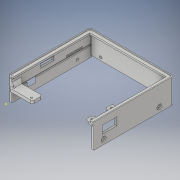
# Autodesk Inventor part: Screen_Top_Open_Back
Saved by Autodesk Inventor 2019 (Build 230136000, 136)
## iProperties
Created: 2020-02-14
Part Number: Screen_Top_Open_Back
Material: Generic
Document SubType Name: Modeling
Designer: zhang
Density: 1 g/cm^3
Appearance: Default
Author: zhang
Autodesk Inventor part; units mm, degrees
note: some values were not read from the file. Chosen so that the rebuilt part matches the saved one: edges of "Chamfer4".
ref_plane "YZ Plane" through (0, 0, 0) normal (1, 0, 0) x (0, 1, 0)
ref_plane "XZ Plane" through (0, 0, 0) normal (0, 1, 0) x (-1, 0, 0)
ref_plane "XY Plane" through (0, 0, 0) normal (0, 0, 1) x (1, 0, 0)
sketch "Sketch1" plane through (0, 0, 0) normal (0, 1, 0) x (-1, 0, 0)
  line L0 (-3, 0) -> (-83, 0)
  line L1 (-86, -3) -> (-86, -83)
  line L2 (-83, -86) -> (-3, -86)
  line L3 (0, -83) -> (0, -3)
  arc A0 (-3, -86) -> (0, -83) centre (-3, -83) ccw
  arc A1 (-86, -83) -> (-83, -86) centre (-83, -83) ccw
  arc A2 (0, -3) -> (-3, 0) centre (-3, -3) ccw
  arc A3 (-83, 0) -> (-86, -3) centre (-83, -3) ccw
  point P0 (0, 0)
  point P1 (-86, -86)
  point P2 (-86, 0)
  point P3 (0, -86)
  dimension "d0" = 86
  dimension "d1" = 86
  dimension "d4" = 3
  constraints: 8 end point, 8 point on circle, 8 point on line, 8 tangent, 4 centre point, 3 equal radius, 2 parallel, 1 horizontal, 1 perpendicular
  measures "d0" distance of point (0, -86) point (-86, -86)
  measures "d1" distance of point (-86, 0) point (-86, -86)
  measures "d4" radius of A0
extrude "Extrusion1" add sketch "Sketch1" along normal blind 25
sketch "Sketch2" plane through (3, 0, 0) normal (0, 0, 1) x (1, 0, 0)
  line L0 (0, 25) -> (80, 25) projected
  line L1 (-2.05, 25) -> (82.05, 25)
  line L2 (82.05, 25) -> (82.05, 24.25)
  line L3 (82.05, 24.25) -> (-2.05, 24.25)
  line L4 (-2.05, 24.25) -> (-2.05, 25)
  line L5 (83, 0) -> (83, 25) projected
  line L6 (0.95, 24.25) -> (79.05, 24.25)
  line L7 (79.05, 24.25) -> (79.05, 22.5)
  line L8 (79.05, 22.5) -> (0.95, 22.5)
  line L9 (0.95, 22.5) -> (0.95, 24.25)
  line L10 (-2.05, 22.5) -> (82.05, 22.5)
  line L11 (82.05, 22.5) -> (82.05, 20.7)
  line L12 (82.05, 20.7) -> (-2.05, 20.7)
  line L13 (-2.05, 20.7) -> (-2.05, 22.5)
  line L14 (-1, 20.7) -> (81, 20.7)
  line L15 (81, 20.7) -> (81, 2)
  line L16 (81, 2) -> (-1, 2)
  line L17 (-1, 2) -> (-1, 20.7)
  line L18 (0, 0) -> (80, 0) projected
  line L19 (-3, 0) -> (-3, 25) projected
  dimension "d5" = 0.75
  dimension "d6" = 84.1
  dimension "d7" = 0.95
  dimension "d8" = 1.75
  dimension "d9" = 3
  dimension "d10" = 3
  dimension "d11" = 1.8
  dimension "d12" = 2
  dimension "d13" = 2
  dimension "d14" = 2
  constraints: 32 end point, 8 parallel, 4 horizontal, 4 perpendicular, 4 point on line, 2 collinear
  measures "d5" distance of L1.end L2.end
  measures "d6" distance of L2.end L3.end
  measures "d7" distance between parallel lines of L5 L2
  measures "d8" distance of L6.end L7.end
  measures "d9" distance between parallel lines of L9 L4
  measures "d10" distance between parallel lines of L2 L7
  measures "d11" distance of L12.end L10.start
  measures "d12" distance between parallel lines of L18 L16
  measures "d13" distance between parallel lines of L19 L17
  measures "d14" distance between parallel lines of L5 L15
extrude "Extrusion2" cut sketch "Sketch2" against normal blind 85.05
sketch "Sketch3" plane through (3, 0, -85.05) normal (0, 0, 1) x (1, 0, 0)
  line L0 (0.95, 22.5) -> (0.95, 24.25) projected
  line L1 (79.05, 24.25) -> (79.05, 22.5) projected
  line L2 (0.95, 24.25) -> (79.05, 24.25)
  line L3 (79.05, 24.25) -> (79.05, 22.5)
  line L4 (79.05, 22.5) -> (0.95, 22.5)
  line L5 (0.95, 22.5) -> (0.95, 24.25)
  point P0 (-3, 0)
  constraints: 8 end point, 2 parallel, 1 horizontal, 1 perpendicular
extrude "Extrusion3" add sketch "Sketch3" along normal blind 3
fillet "Fillet1" radius 2 2 edges at (85.05, 24.625, -85.05) (0.95, 24.625, -85.05)
sketch "Sketch4" plane through (0, 0, -83) normal (-1, 0, 0) x (0, 0, 1)
  line L0 (7.95, 14.25) -> (21.95, 14.25)
  line L1 (21.95, 14.25) -> (21.95, 12.25)
  line L2 (21.95, 12.25) -> (7.95, 12.25)
  line L3 (7.95, 12.25) -> (7.95, 14.25)
  line L4 (82.1903, 24.25) -> (-0.05, 24.25) projected
  line L5 (-2.05, 24.25) -> (-2.05, 25) projected
  point P0 (83, 0)
  dimension "d20" = 14
  dimension "d21" = 2
  dimension "d22" = 10
  dimension "d23" = 10
  constraints: 8 end point, 2 parallel, 1 horizontal, 1 perpendicular
  measures "d20" distance of L0.start L0.end
  measures "d21" distance of L2.end L0.start
  measures "d22" distance between parallel lines of L4 L0
  measures "d23" distance between parallel lines of L3 L5
extrude "Extrusion4" cut sketch "Sketch4" against normal up to next
sketch "Sketch5" plane through (0, 12.25, -61.05) normal (0, 1, 0) x (1, 0, 0)
  line L0 (0, 0) -> (0, 14) projected
  line L1 (0, 14) -> (-15, 14)
  line L2 (-15, 14) -> (-15, 0)
  line L3 (-15, 0) -> (0, 0)
  line L4 (0, 0) -> (0, 14)
  circle A0 centre (-15, 7) radius 18.801
  point P0 (0, -61.05)
  point P1 (2, 14)
  dimension "d26" = 15
  dimension "d27" = 14
  constraints: 8 end point, 2 parallel, 1 centre point, 1 horizontal, 1 midpoint, 1 perpendicular
  measures "d26" distance of L3.end L2.end
  measures "d27" distance of L2.end L1.end
extrude "Extrusion5" cut sketch "Sketch5" along normal blind 2 contours L3 L2 L1 L0 | A0
sketch "Sketch6" plane through (3, 0, 0) normal (0, 0, 1) x (1, 0, 0)
  line L0 (83, 0) -> (83, 25) projected
  line L1 (-3, 0) -> (83, 0)
  line L2 (83, 0) -> (83, 25)
  line L3 (83, 25) -> (-3, 25)
  line L4 (-3, 25) -> (-3, 0)
  constraints: 8 end point, 2 parallel, 1 horizontal, 1 perpendicular
extrude "Extrusion6" cut sketch "Sketch6" against normal blind 4
sketch "Sketch7" plane through (86, 0, -3) normal (1, 0, 0) x (0, 0, -1)
  circle A0 centre (11, 5) radius 1.3
  line L0 (1, 25) -> (1, 0) projected
  line L1 (1, 25) -> (80, 25) projected
  line L2 (1, 0) -> (80, 0) projected
  circle A1 centre (68, 5) radius 1.3
  line L3 (83, 0) -> (83, 25) projected
  dimension "d35" = 2.6
  dimension "d64" = 10
  dimension "d89" = 5
  dimension "d98" = 2.6
  dimension "d99" = 5
  dimension "d100" = 15
  constraints: 2 centre point
  measures "d35" diameter of A0
  measures "d64" distance from line of A0.centre L0
  measures "d89" distance from line of L2 A0.centre
  measures "d98" diameter of A1
  measures "d99" distance from line of L2 A1.centre
  measures "d100" distance from line of L3 A1.centre
extrude "Extrusion7" cut sketch "Sketch7" against normal through all
sketch "Sketch8" plane through (86, 0, -3) normal (1, 0, 0) x (0, 0, -1)
  circle A0 centre (11, 5) radius 1.3 projected
  circle A1 centre (11, 5) radius 2.5
  circle A2 centre (68, 5) radius 1.3 projected
  circle A3 centre (68, 5) radius 2.5
  point P0 (-3, 0)
  dimension "d40" = 5
  dimension "d101" = 5
  constraints: 2 centre point, 2 coincident
  measures "d40" diameter of A1
  measures "d101" diameter of A3
extrude "Extrusion8" cut sketch "Sketch8" against normal blind 1
sketch "Sketch9" plane through (0, 0, -83) normal (-1, 0, 0) x (0, 0, 1)
  circle A0 centre (69, 5) radius 1.3 projected
  circle A1 centre (69, 5) radius 2.5
  circle A2 centre (12, 5) radius 1.3 projected
  circle A3 centre (12, 5) radius 2.5
  point P0 (83, 0)
  dimension "d43" = 5
  dimension "d102" = 5
  constraints: 2 centre point, 2 coincident
  measures "d43" diameter of A1
  measures "d102" diameter of A3
extrude "Extrusion9" cut sketch "Sketch9" against normal blind 1 contours A1 | A2 | A3
fillet "Fillet2" radius 2 2 edges at (85.05, 21.6, -85.05) (0.95, 21.6, -85.05)
sketch "Sketch13" plane through (3, 0, -4) normal (0, 0, 1) x (1, 0, 0)
  line L0 (-2.05, 12.15) -> (-1, 12.15)
  line L1 (-1, 12.15) -> (-1, 10.65)
  line L2 (-1, 10.65) -> (-2.05, 10.65)
  line L3 (-2.05, 10.65) -> (-2.05, 12.15)
  line L4 (-2.05, 20.7) -> (-1, 20.7) projected
  line L5 (-2.05, 22.5) -> (-2.05, 20.7) projected
  line L6 (-1, 20.7) -> (-1, 2) projected
  line L7 (-3, 25) -> (-2.05, 25) projected
  point P0 (-3, 0)
  dimension "d70" = 1.5
  dimension "d86" = 14.35
  constraints: 8 end point, 2 collinear, 2 parallel, 1 horizontal, 1 perpendicular
  measures "d70" distance of L2.end L0.start
  measures "d86" distance between parallel lines of L2 L7
extrude "Extrusion13" cut sketch "Sketch13" against normal blind 80.5
chamfer "Chamfer2" distance 2 angle 45 3 edges at (0, 14.25, -68.05) (0, 13.25, -56.7151) (0, 13.25, -79.3849)
sketch "Sketch14" plane through (0, 0, -83) normal (-1, 0, 0) x (0, 0, 1)
  line L0 (35.95, 20.25) -> (49.95, 20.25)
  line L1 (49.95, 20.25) -> (49.95, 16.25)
  line L2 (49.95, 16.25) -> (35.95, 16.25)
  line L3 (35.95, 16.25) -> (35.95, 20.25)
  line L4 (-2.05, 24.25) -> (-2.05, 25) projected
  line L5 (0, 25) -> (79, 25) projected
  point P0 (83, 0)
  dimension "d77" = 4
  dimension "d78" = 14
  dimension "d81" = 8.75
  dimension "d82" = 52
  constraints: 8 end point, 2 parallel, 1 horizontal, 1 perpendicular
  measures "d77" distance of L0.end L1.end
  measures "d78" distance of L0.start L0.end
  measures "d81" distance between parallel lines of L5 L2
  measures "d82" distance between parallel lines of L1 L4
extrude "Extrusion14" cut sketch "Sketch14" against normal blind 10
sketch "Sketch15" plane through (3, 0, -4) normal (0, 0, 1) x (1, 0, 0)
  line L0 (81, 2) -> (81, 20.7) projected
  line L1 (81, 2) -> (-1, 2)
  line L2 (-1, 2) -> (-1, 0)
  line L3 (-1, 0) -> (81, 0)
  line L4 (81, 0) -> (81, 2)
  line L5 (-1, 10.65) -> (-1, 2) projected
  line L6 (83, 0) -> (-3, 0) projected
  constraints: 8 end point, 2 collinear, 2 parallel, 1 horizontal, 1 perpendicular
extrude "Extrusion15" cut sketch "Sketch15" against normal up to next
sketch "Sketch16" plane through (83, 25, -86) normal (0, 0, -1) x (-1, 0, 0)
  circle A0 centre (71, -20) radius 1.3
  circle A1 centre (9, -20) radius 1.3
  line L0 (81, -23) -> (81, -25) projected
  line L1 (-1, -25) -> (-1, -23) projected
  line L2 (83, -25) -> (81, -25) projected
  line L3 (-1, -25) -> (-3, -25) projected
  dimension "d90" = 2.6
  dimension "d91" = 2.6
  dimension "d92" = 10
  dimension "d93" = 10
  dimension "d94" = 5
  dimension "d95" = 5
  constraints: 2 centre point
  measures "d90" diameter of A0
  measures "d91" diameter of A1
  measures "d92" distance from line of A0.centre L0
  measures "d93" distance from line of L1 A1.centre
  measures "d94" distance from line of L2 A0.centre
  measures "d95" distance from line of L3 A1.centre
extrude "Extrusion16" cut sketch "Sketch16" against normal blind 10
sketch "Sketch17" plane through (0, 0, -83) normal (-1, 0, 0) x (0, 0, 1)
  point P0 (83, 0)
sketch "Sketch18" plane through (84, 0, -4) normal (-1, 0, 0) x (0, 0, 1)
  line L0 (-2, 18.7) -> (-10, 18.7)
  line L1 (-10, 18.7) -> (-10, 20.7)
  line L2 (-10, 20.7) -> (-2, 20.7)
  line L3 (-2, 20.7) -> (-2, 18.7)
  line L4 (0, 20.7) -> (-79.05, 20.7) projected
  line L5 (0, 25) -> (0, 0) projected
  line L6 (-22, 20.7) -> (-30, 20.7)
  line L7 (-30, 20.7) -> (-30, 18.7)
  line L8 (-30, 18.7) -> (-22, 18.7)
  line L9 (-22, 18.7) -> (-22, 20.7)
  point P0 (4, 0)
  dimension "d103" = 8
  dimension "d104" = 2
  dimension "d105" = 8
  dimension "d106" = 12
  dimension "d107" = 2
  dimension "d155" = 2
  constraints: 16 end point, 4 parallel, 2 horizontal, 2 perpendicular, 1 collinear, 1 point on line
  measures "d103" distance of L1.end L2.end
  measures "d104" distance of L0.end L1.end
  measures "d105" distance of L8.end L7.end
  measures "d106" distance from line of L8.end L1
  measures "d107" distance of L6.end L7.end
  measures "d155" distance between parallel lines of L5 L3
extrude "Extrusion17" add sketch "Sketch18" along normal blind 9
fillet "Fillet3" radius 3 4 edges at (75, 19.7, -26) (75, 19.7, -34) (75, 19.7, -6) (75, 19.7, -14)
sketch "Sketch19" plane through (84, 18.7, -14) normal (0, -1, 0) x (1, 0, 0)
  circle A0 centre (-5.85, 4.15) radius 1
  circle A1 centre (-5.85, -15.85) radius 1
  line L0 (2, 10) -> (0, 10) projected
  line L1 (0, 10) -> (0, -71.8284) projected
  point P0 (-84, 14)
  dimension "d111" = 2
  dimension "d112" = 2
  dimension "d113" = 5.85
  dimension "d114" = 5.85
  dimension "d115" = 5.85
  dimension "d116" = 20
  constraints: 2 centre point
  measures "d111" diameter of A0
  measures "d112" diameter of A1
  measures "d113" distance from line of A0.centre L0
  measures "d114" distance from line of L1 A0.centre
  measures "d115" distance from line of L1 A1.centre
  measures "d116" distance of A0.centre A1.centre
extrude "Extrusion18" cut sketch "Sketch19" against normal blind 12
sketch "Sketch20" plane through (84, 0, -85.8284) normal (-1, 0, 0) x (0, 0, 1)
  line L0 (73.2284, 10) -> (58.2284, 10)
  line L1 (58.2284, 10) -> (58.2284, 18)
  line L2 (58.2284, 18) -> (73.2284, 18)
  line L3 (73.2284, 18) -> (73.2284, 10)
  line L4 (81.8284, 25) -> (81.8284, 0) projected
  line L5 (81.8284, 0) -> (2.8284, 0) projected
  point P0 (85.8284, 0)
  dimension "d119" = 15
  dimension "d121" = 10
  dimension "d122" = 8
  dimension "d156" = 8.6
  constraints: 8 end point, 2 parallel, 1 horizontal, 1 perpendicular
  measures "d119" distance of L1.end L2.end
  measures "d121" distance between parallel lines of L5 L0
  measures "d122" distance of L2.end L0.start
  measures "d156" distance between parallel lines of L4 L3
extrude "Extrusion19" cut sketch "Sketch20" against normal blind 12
sketch "Sketch21" plane through (2, 0, -4) normal (1, 0, 0) x (0, 0, -1)
  line L0 (0, 12.15) -> (80.5, 12.15) projected
  line L1 (7, 12.15) -> (-3, 12.15)
  line L2 (-3, 12.15) -> (-3, 15.15)
  line L3 (-3, 15.15) -> (7, 15.15)
  line L4 (7, 15.15) -> (7, 12.15)
  line L5 (0, 0) -> (0, 25) projected
  point P0 (-4, 0)
  dimension "d125" = 10
  dimension "d126" = 3
  dimension "d127" = 7
  constraints: 8 end point, 2 parallel, 1 horizontal, 1 perpendicular, 1 point on line
  measures "d125" distance of L2.end L3.end
  measures "d126" distance of L1.end L2.end
  measures "d127" distance between parallel lines of L5 L4
extrude "Extrusion20" add sketch "Sketch21" along normal blind 24
chamfer "Chamfer3" distance 3 angle 45 1 edges at (2, 13.65, -11)
chamfer "Chamfer4" distance 3 angle 45 1 edges at (2, 15.15, -7.5)
fillet "Fillet4" radius 2 1 edges at (2, 13.65, -1)
fillet "Fillet5" radius 2 2 edges at (26, 13.65, -1) (26, 13.65, -11)
sketch "Sketch22" plane through (0.95, 12.15, -84.5) normal (0, -1, 0) x (1, 0, 0)
  circle A0 centre (3.65, 80.96) radius 1
  circle A1 centre (21.65, 80.96) radius 1
  line L0 (1.05, -1.3284) -> (1.05, 80.5) projected
  line L1 (3.05, 83.5) -> (23.05, 83.5) projected
  point P0 (-0.95, 84.5)
  dimension "d138" = 2
  dimension "d139" = 2
  dimension "d140" = 2.6
  dimension "d141" = 2.54
  dimension "d142" = 2.54
  dimension "d143" = 18
  constraints: 2 centre point
  measures "d138" diameter of A0
  measures "d139" diameter of A1
  measures "d140" distance from line of A0.centre L0
  measures "d141" distance from line of L1 A0.centre
  measures "d142" distance from line of L1 A1.centre
  measures "d143" distance of A1.centre A0.centre
extrude "Extrusion21" cut sketch "Sketch22" against normal blind 5
sketch "Sketch23" plane through (2, 0, -4) normal (1, 0, 0) x (0, 0, -1)
  line L0 (24.35, 5.9) -> (15.6, 5.9)
  line L1 (15.6, 5.9) -> (15.6, 10.65)
  line L2 (15.6, 10.65) -> (24.35, 10.65)
  line L3 (24.35, 10.65) -> (24.35, 5.9)
  line L4 (0, 0) -> (0, 25) projected
  line L5 (0, 10.65) -> (80.5, 10.65) projected
  point P0 (-4, 0)
  dimension "d146" = 8.75
  dimension "d147" = 4.75
  dimension "d148" = 24.35
  constraints: 8 end point, 2 parallel, 1 collinear, 1 horizontal, 1 perpendicular
  measures "d146" distance of L1.end L2.end
  measures "d147" distance of L0.end L1.end
  measures "d148" distance between parallel lines of L4 L3
extrude "Extrusion22" cut sketch "Sketch23" against normal blind 5
chamfer "Chamfer5" distance 2 angle 45 3 edges at (0, 5.9, -23.975) (0, 8.275, -19.6) (0, 8.275, -28.35)
body "Solid1"
